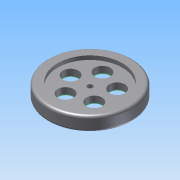
# Autodesk Inventor part: 바퀴
Saved by Autodesk Inventor 2011 (Build 150239000, 239)
## iProperties
Created: 2019-04-02
Part Number: 바퀴
Document SubType Name: Modeling
Designer: User
Density: 1 g/cm^3
Author: User
Autodesk Inventor part; units mm, degrees
ref_plane "YZ Plane" through (0, 0, 0) normal (1, 0, 0) x (0, 1, 0)
ref_plane "XZ Plane" through (0, 0, 0) normal (0, 1, 0) x (-1, 0, 0)
ref_plane "XY Plane" through (0, 0, 0) normal (0, 0, 1) x (1, 0, 0)
sketch "스케치2" plane through (0, 0, 0) normal (0, 0, 1) x (1, 0, 0)
  circle A0 centre (0, 0) radius 32.5
  circle A1 centre (0, 0) radius 25
  circle A2 centre (0, 0) radius 3
  circle A3 centre (-15, 0) radius 6
  circle A4 centre (-4.6353, -14.2658) radius 6
  circle A5 centre (12.1353, -8.8168) radius 6
  circle A6 centre (12.1353, 8.8168) radius 6
  circle A7 centre (-4.6353, 14.2658) radius 6
  circle A8 centre (0, 0) radius 2
  dimension "d0" = 65
  dimension "d3" = 50
  dimension "d4" = 6
  dimension "d6" = 12
  dimension "d7" = 15
  dimension "d10" = 360
  dimension "d12" = 4
  constraints: 9 centre point, 3 coincident, 11 other
  measures "d0" diameter of A0
  measures "d3" diameter of A1
  measures "d4" diameter of A2
  measures "d6" diameter of A3
  measures "d7" distance of A2.centre A3.centre
  measures "d12" diameter of A8
extrude "돌출1" add sketch "스케치2" along normal blind 11 contours A0 | A1 | A2 | A3 | A4 | A5 | A6 | A7 | A8
extrude "돌출2" cut sketch "스케치2" along normal blind 3 contours A1
extrude "돌출3" cut sketch "스케치2" along normal blind 11 contours A3 | A4 | A5 | A6 | A7 | A8
sketch "스케치3" plane through (0, 0, 11) normal (0, 0, 1) x (1, 0, 0)
  circle A0 centre (0, 0) radius 2 projected
  circle A1 centre (-4.6353, 14.2658) radius 6 projected
  circle A2 centre (12.1353, 8.8168) radius 6 projected
  circle A3 centre (12.1353, -8.8168) radius 6 projected
  circle A4 centre (-4.6353, -14.2658) radius 6 projected
  circle A5 centre (-15, 0) radius 6 projected
  circle A6 centre (0, 0) radius 32.5 projected
  circle A7 centre (0, 0) radius 25
  dimension "d17" = 50
  constraints: 1 centre point, 1 coincident
  measures "d17" diameter of A7
extrude "돌출4" cut sketch "스케치3" against normal blind 3 contours A7
chamfer "모따기1" distance 0.5 angle 45 1 edges at (-2, 0, 0)
fillet "모깎기1" radius 2 1 edges at (-32.5, 0, 11)
fillet "모깎기2" radius 2 1 edges at (-32.5, 0, 0)
sketch "스케치4" plane through (0, 0, 3) normal (0, 0, -1) x (-1, 0, 0)
  circle A0 centre (4.6353, 14.2658) radius 6 projected
  circle A1 centre (-12.1353, 8.8168) radius 6 projected
  circle A2 centre (-12.1353, -8.8168) radius 6 projected
  circle A3 centre (4.6353, -14.2658) radius 6 projected
  circle A4 centre (15, 0) radius 6 projected
  circle A5 centre (0, 0) radius 3 projected
  circle A6 centre (0, 0) radius 25 projected
